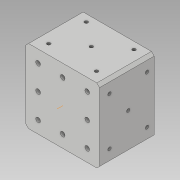
# Autodesk Inventor part: cube_square_tube
Saved by Autodesk Inventor 2017 (Build 210142000, 142)
## iProperties
Part Number: cube_square_tube
Material: Aluminium 6061
Document SubType Name: Modeling
Designer: Max
Density: 2.7 g/cm^3
Appearance: Vorgabe
Mass: 103.061 g
Surface Area: 193.007 cm^2
Volume: 38.1708 cm^3
Author: Max
Autodesk Inventor part; units mm, degrees
ref_plane "YZ Plane" through (0, 0, 0) normal (1, 0, 0) x (0, 1, 0)
ref_plane "XZ Plane" through (0, 0, 0) normal (0, 1, 0) x (-1, 0, 0)
ref_plane "XY Plane" through (0, 0, 0) normal (0, 0, 1) x (1, 0, 0)
sketch "Skizze1" plane through (0, 0, 0) normal (0, 1, 0) x (-1, 0, 0)
  line L0 (-27, 27) -> (27, 27)
  line L1 (27, 27) -> (27, -27)
  line L2 (27, -27) -> (-27, -27)
  line L3 (-27, -27) -> (-27, 27)
  line L4 (-27, 27) -> (27, -27) construction
  line L5 (27, 27) -> (-27, -27) construction
  point P0 (0, 0)
  dimension "d0" = 54
  dimension "d1" = 54
  constraints: 12 end point, 2 midpoint, 2 parallel, 1 horizontal, 1 perpendicular
  measures "d0" distance of L1.end L2.end
  measures "d1" distance of L0.end L1.end
extrude "Extrusion1" add sketch "Skizze1" along normal blind 40
sketch "Skizze2" plane through (0, 40, 0) normal (0, 1, 0) x (1, 0, 0)
  line L0 (23, -23) -> (-23, -23)
  line L1 (-23, -23) -> (-23, 23)
  line L2 (-23, 23) -> (23, 23)
  line L3 (23, 23) -> (23, -23)
  line L4 (23, -23) -> (-23, 23) construction
  line L5 (-23, -23) -> (23, 23) construction
  line L6 (-27, -27) -> (27, -27) projected
  line L7 (27, -27) -> (27, 27) projected
  line L8 (27, 27) -> (-27, 27) projected
  line L9 (-27, 27) -> (-27, -27) projected
  point P0 (0, 0)
  dimension "d4" = 4
  dimension "d5" = 4
  constraints: 12 end point, 2 midpoint, 2 parallel, 1 horizontal, 1 perpendicular
  measures "d4" distance between parallel lines of L8 L2
  measures "d5" distance between parallel lines of L9 L1
extrude "Extrusion2" cut sketch "Skizze2" against normal blind 35 contours L0 L1 L2 L3
fillet "Rundung1" radius 4 4 edges at (-23, 22.5, -23) (23, 22.5, -23) (-23, 22.5, 23) (23, 22.5, 23)
sketch "Skizze3" plane through (0, 0, 0) normal (0, -1, 0) x (1, 0, 0)
  line L0 (-18, 18) -> (18, 18)
  line L1 (18, 18) -> (18, -18)
  line L2 (18, -18) -> (-18, -18)
  line L3 (-18, -18) -> (-18, 18)
  line L4 (-18, 18) -> (18, -18) construction
  line L5 (18, 18) -> (-18, -18) construction
  line L6 (18, 0) -> (-18, 0) construction
  line L7 (0, 18) -> (0, -18) construction
  point P0 (0, 0)
  dimension "d9" = 36
  dimension "d10" = 36
  constraints: 16 end point, 6 midpoint, 2 parallel, 1 horizontal, 1 perpendicular
  measures "d9" distance of L0.end L1.end
  measures "d10" distance of L1.end L2.end
hole "Bohrung1" at (18, 0, 18) at (18, 0, 0) at (18, 0, -18) at (0, 0, -18) at (-18, 0, -18) at (-18, 0, 0) at (-18, 0, 18) at (0, 0, 18) direction (0, 1, 0) diameter 3.4 end through all clearance for "Inbusschraube ISO 4762" size "M3" standard "ISO"
sketch "Skizze5" plane through (27, 0, 27) normal (1, 0, 0) x (0, 0, -1)
  line L0 (9.5, 7.25) -> (44.5, 7.25)
  line L1 (44.5, 7.25) -> (44.5, 34.75)
  line L2 (44.5, 34.75) -> (9.5, 34.75)
  line L3 (9.5, 34.75) -> (9.5, 7.25)
  line L4 (9.5, 7.25) -> (44.5, 34.75) construction
  line L5 (44.5, 7.25) -> (9.5, 34.75) construction
  line L6 (54, 0) -> (0, 0) projected
  line L7 (54, 0) -> (54, 40) projected
  line L8 (0, 40) -> (54, 40) projected
  line L9 (0, 0) -> (0, 40) projected
  point P0 (27, 0)
  point P1 (27, 21)
  dimension "d18" = 9.5
  dimension "d21" = 35
  dimension "d29" = 27.5
  dimension "d30" = 54
  dimension "d46" = 21
  dimension "d47" = 27
  constraints: 12 end point, 2 midpoint, 2 parallel, 1 horizontal, 1 perpendicular
  measures "d18" distance between parallel lines of L7 L1
  measures "d21" distance of L1.end L2.end
  measures "d29" distance of L2.end L0.start
  measures "d30" distance of L6.start L6.end
  measures "d46" vertical distance of L6.start point (27, 21)
  measures "d47" distance from line of L9 point (27, 21)
hole "Bohrung2" at (27, 34.75, 17.5) at (27, 21, 0) at (27, 34.75, -17.5) at (27, 7.25, -17.5) at (27, 7.25, 17.5) direction (-1, 0, 0) diameter 2.459 depth 8.8 tip angle 118 thread size "M3x0.5" class "6H" standard "ISO Metric profile"
ref_plane "Arbeitsebene1" through (27, 40, -27) normal (-0.7071068, 0, -0.7071068) x (0, -1, 0)
mirror "Spiegeln1" about plane through (27, 40, -27) normal (-0.7071068, 0, -0.7071068) of "Bohrung2"
ref_plane "Arbeitsebene2" through (27, 40, 27) normal (0.7071068, 0, -0.7071068) x (0, -1, 0)
mirror "Spiegeln2" about plane through (27, 40, 27) normal (0.7071068, 0, -0.7071068) of "Bohrung2", "Spiegeln1"
chamfer "Fase3" distance 2 angle 45 4 edges at (27, 20, 27) (27, 20, -27) (-27, 20, -27) (-27, 20, 27)
equation "\"d18\" = -0.5 * d21 + 0.5 * d30"
equation "\"d47\" = 0.5 * d30"
